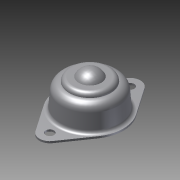
# Autodesk Inventor part: Ball_and_Socket
Saved by Autodesk Inventor 2011 SP2 (Build 150309200, 309)
## iProperties
Created: 2015-10-31
Part Number: Ball_and_Socket
Document SubType Name: Modeling
Designer: Ernest
Density: 1 g/cm^3
Mass: 8.73385 g
Surface Area: 30.4562 cm^2
Volume: 8.73385 cm^3
Author: Ernest
Autodesk Inventor part; units mm, degrees
ref_plane "YZ Plane" through (0, 0, 0) normal (1, 0, 0) x (0, 1, 0)
ref_plane "XZ Plane" through (0, 0, 0) normal (0, 1, 0) x (-1, 0, 0)
ref_plane "XY Plane" through (0, 0, 0) normal (0, 0, 1) x (1, 0, 0)
sketch "Sketch1" plane through (0, 0, 0) normal (0, 0, 1) x (1, 0, 0)
  line L0 (0, 0) -> (15.7399, 0)
  line L1 (0, 0) -> (0, 8.3)
  line L2 (0, 8.3) -> (0, 11.9)
  line L3 (0, 11.9) -> (0, 13.9)
  line L4 (5.4046, 13.9) -> (7.9673, 13.9)
  line L5 (13.75, 8.3) -> (14.25, 1.5)
  arc A0 (14.25, 1.5) -> (15.7399, 0) centre (15.87, 1.6191) ccw
  arc A1 (13.75, 8.3) -> (10, 11.9) centre (9.8734, 8.015) ccw
  arc A2 (10, 11.9) -> (7.9673, 13.9) centre (7.9673, 11.867) ccw
  line L6 (0, 13.9) -> (0, 17.3)
  arc A3 (5.4046, 13.9) -> (0, 17.3) centre (0, 11.3044) ccw
  constraints: 14 end point, 8 point on circle, 4 centre point, 3 tangent, 2 perpendicular, 1 horizontal, 1 point on line
revolve "Revolution1" add sketch "Sketch1" angle 360 about axis through (0, 0, 0) along (0, 1, 0)
sketch "Sketch2" plane through (0, 0, 0) normal (0, -1, 0) x (1, 0, 0)
  circle A0 centre (0, 0) radius 15.7399 projected
  circle A1 centre (0, 19.45) radius 2
  circle A2 centre (0, -19.45) radius 2
  line L0 (-13.2082, 9.1184) -> (-4.1147, 22.2906)
  line L1 (-13.2082, -9.1184) -> (-4.1147, -22.2906)
  line L2 (4.1147, -22.2906) -> (13.2082, -9.1184)
  line L3 (13.2082, 9.1184) -> (4.1147, 22.2906)
  line L4 (0, -24.45) -> (0, 24.45) construction
  arc A3 (-4.1147, -22.2906) -> (4.1147, -22.2906) centre (0, -19.45) ccw
  arc A4 (13.2082, -9.1184) -> (13.2082, 9.1184) centre (0, 0) ccw
  arc A5 (-13.2082, 9.1184) -> (-13.2082, -9.1184) centre (0, 0) ccw
  arc A6 (4.1147, 22.2906) -> (-4.1147, 22.2906) centre (0, 19.45) ccw
  dimension "d11" = 4
  dimension "d12" = 4
  dimension "d13" = 34.9
  dimension "d14" = 19.45
  constraints: 10 end point, 10 point on circle, 8 tangent, 6 centre point, 3 coincident, 1 midpoint, 1 parallel, 1 point on line, 1 vertical
  measures "d11" diameter of A2
  measures "d12" diameter of A1
  measures "d14" distance of A0.centre A2.centre
extrude "Extrusion1" add sketch "Sketch2" along normal blind 0.9 contours A0 | L0 A6 L3 A4 L2 A3 L1 A5
body "Solid1"
